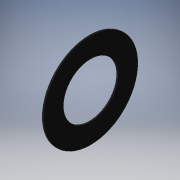
# Autodesk Inventor part: 6000DDU Shield1
Saved by Autodesk Inventor 2019 (Build 230136000, 136)
## iProperties
Created: 2023-07-21
Part Number: 6000DDU Shield1
Material: Generic
Catalog Web Link: www.cadenas.de
Description: contact_sealed_type_dd_ddu_S1-NSK
Vendor: NSK_RB
Document SubType Name: Modeling
Designer: psAdmin
Manufacturer: NSK_RB
Mass: 0.0769013 g
Surface Area: 5.88644 cm^2
Volume: 0.0769013 cm^3
Density: 1 g/cm^3
Appearance: PSOLRGB-128-128-128
Category: PARTsolutions
Company: NSK_RB
Title: 6000DDU Shield1
Author: Cadenas PARTsolutions
Comments: NSK
PSOL_IDENT_0: {$CADENAS_DATA/23d-libs/nsk_rb/roller_bearings/deep_groove_bb/single_row_dgbb/contact_sealed_type_dd
PSOL_IDENT_1: _ddu_4_s1.prj},193 {VTYP=3D},{NB=6000DDU Shield1},{LINA=6000DDU Shield1},{NN=contact_sealed_type_dd_
PSOL_IDENT_2: ddu_S1},{DATE=15.09.2022 00:32:48},{GEOMDATE=18.05.2018 11:37:34},{VERSION=},{LINEID=30},{WBVAR=},{W
PSOL_IDENT_3: BNUMERIC=}  {NB=6000DDU Shield1},{LINA=6000DDU Shield1},{KT=DUMMY},{IDNR=},{STAN=Standard},{ORDER=60
PSOL_IDENT_4: 00DDU},{SD=10},{X=10},{DI1=14.57},{DI2=13.2},{SDE1=21.50},{SDE2=23.00},{D=26},{DD=26},{B=8},{R=0.3},
PSOL_IDENT_5: {CR1=4550},{COR1=1970},{CR2=465},{COR2=201},{FO=12.4},{LG=22000},{A=1.35},{BB=0.87},{DD1=24.50},{RO=
PSOL_IDENT_6: 0.20},{RN=0.3},{DD2=28.7},{F=0.84},{DAM1=12.0},{DA1=13.0},{DA2=24.0},{RA=0.3},{DX=29.4},{CY=1.9},{MA
PSOL_IDENT_7: SS=0.018},{SC=1}
NB: 6000DDU Shield1
NN: contact_sealed_type_dd_ddu_S1
NT: NSK
NBSYN: $ORDER. Shield1
LINA: 6000DDU Shield1
CATALOG: NSK Rolling Bearing
STAN: Standard
ORDER: 6000DDU
SD: 10
X: 10
DI1: 14.57
DI2: 13.2
SDE1: 21.5
SDE2: 23
D: 26
DD: 26
B: 8
R: 0.3
CR1: 4550
COR1: 1970
CR2: 465
COR2: 201
FO: 12.4
LG: 22000
A: 1.35
BB: 0.87
DD1: 24.5
RO: 0.2
RN: 0.3
DD2: 28.7
F: 0.84
DAM1: 12
DA1: 13
DA2: 24
RA: 0.3
DX: 29.4
CY: 1.9
MASS: 0.018
SC: 1
SUPPLIER: NSK_RB
ARTICLENO: 6000DDU Shield1
BOMINFO: 6000DDU Shield1
CREATOR: CADENAS GmbH
Autodesk Inventor part; units mm, degrees
ref_plane "YZ Plane" through (0, 0, 0) normal (1, 0, 0) x (0, 1, 0)
ref_plane "XZ Plane" through (0, 0, 0) normal (0, 1, 0) x (-1, 0, 0)
ref_plane "XY Plane" through (0, 0, 0) normal (0, 0, 1) x (1, 0, 0)
sketch "Sketch_1" plane through (0, 0, 0) normal (0, 0, 1) x (1, 0, 0)
  line L0 (0.276, 0) -> (0, 0)
  line L1 (0, 6.6) -> (0.276, 6.6)
  line L2 (0.276, 6.6) -> (0.276, 11.5)
  line L3 (0.276, 11.5) -> (0, 11.5)
  line L4 (0, 11.5) -> (0, 6.6)
  constraints: 10 end point
revolve "Revolution1" add sketch "Sketch_1" angle 360 about axis through (0.276, 0, 0) along (1, 0, 0)
ref_plane "ip_cst_4_s1_XY" through (0, 0, 0) normal (1, 0, 0) x (0, 0, -1)
ref_plane "ip_cst_4_s1_YZ" through (0, 0, 0) normal (0, 0, -1) x (0, 1, 0)
ref_plane "ip_cst_4_s1_ZX" through (0, 0, 0) normal (0, 1, 0) x (1, 0, 0)
body "Solid1"
